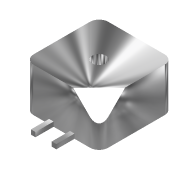
# Autodesk Inventor part: 01_Body
Saved by Autodesk Inventor 2016 (Build 200138000, 138)
## iProperties
Created: 2017-03-03
Part Number: 01_Body
Material: Generisch
Document SubType Name: Modeling
Designer: diederichbenedict
Density: 1 g/cm^3
Appearance: Chrom - poliert
Author: diederichbenedict
Autodesk Inventor part; units mm, degrees
ref_plane "YZ Plane" through (0, 0, 0) normal (1, 0, 0) x (0, 1, 0)
ref_plane "XZ Plane" through (0, 0, 0) normal (0, 1, 0) x (-1, 0, 0)
ref_plane "XY Plane" through (0, 0, 0) normal (0, 0, 1) x (1, 0, 0)
sketch "Skizze1" plane through (0, 0, 0) normal (0, 0, 1) x (1, 0, 0)
  line L0 (-4.1, 4.1) -> (4.1, 4.1)
  line L1 (4.1, 4.1) -> (4.1, -4.1)
  line L2 (4.1, -4.1) -> (-4.1, -4.1)
  line L3 (-4.1, -4.1) -> (-4.1, 4.1)
  line L4 (-4.1, 4.1) -> (4.1, -4.1) construction
  line L5 (4.1, 4.1) -> (-4.1, -4.1) construction
  point P0 (0, 0)
  dimension "d0" = 8.2
  dimension "d1" = 8.2
  constraints: 12 end point, 2 midpoint, 2 parallel, 1 horizontal, 1 perpendicular
  measures "d0" distance of L1.end L2.end
  measures "d1" distance of L0.end L1.end
extrude "Extrusion1" add sketch "Skizze1" along normal blind 4.8
sketch "Skizze3" plane through (0, 0, 0) normal (0, 0, -1) x (-1, 0, 0)
  line L0 (4.1, 4.1) -> (-4.1, 4.1) projected
  line L1 (-4.1, 4.1) -> (-4.1, -4.1) projected
  line L2 (-4.1, -4.1) -> (4.1, -4.1) projected
  line L3 (4.1, -4.1) -> (4.1, 4.1) projected
  circle A0 centre (0, 0) radius 3.5
  dimension "d7" = 7
  constraints: 1 centre point, 1 coincident
  measures "d7" diameter of A0
extrude "Extrusion3" cut sketch "Skizze3" against normal blind 2.5 contours A0
fillet "Rundung1" radius 1 4 edges at (4.1, -4.1, 2.4) (-4.1, -4.1, 2.4) (-4.1, 4.1, 2.4) (4.1, 4.1, 2.4)
sketch "Skizze4" plane through (0, 0, 4.8) normal (0, 0, 1) x (1, 0, 0)
  circle A0 centre (0, 0) radius 3.5 projected
  circle A1 centre (0, 0) radius 0.75
  dimension "d11" = 1.5
  constraints: 1 centre point, 1 coincident
  measures "d11" diameter of A1
extrude "Extrusion4" cut sketch "Skizze4" against normal blind 2.5 contours A1
sketch "Skizze5" plane through (-3.1, -4.1, 0) normal (0, -1, 0) x (1, 0, 0)
  line L0 (3.1, 0) -> (3.1, 4.8)
  line L1 (2.35, 4.8) -> (3.85, 4.8) projected
  line L2 (6.2, 0) -> (0, 0) projected
  line L3 (2.2019, 0) -> (1.7019, 0)
  line L4 (1.7019, 0) -> (1.7019, 0.5)
  line L5 (1.7019, 0.5) -> (2.2019, 0.5)
  line L6 (2.2019, 0.5) -> (2.2019, 0)
  line L7 (3.9981, 0) -> (4.4981, 0)
  line L8 (4.4981, 0) -> (4.4981, 0.5)
  line L9 (4.4981, 0.5) -> (3.9981, 0.5)
  line L10 (3.9981, 0.5) -> (3.9981, 0)
  dimension "d14" = 0.5
  dimension "d15" = 0.5
  constraints: 18 end point, 4 symmetric about line, 2 parallel, 1 horizontal, 1 midpoint, 1 perpendicular, 1 point on line
  measures "d14" distance of L4.end L5.end
  measures "d15" distance of L3.end L4.end
extrude "Extrusion5" add sketch "Skizze5" along normal blind 2
